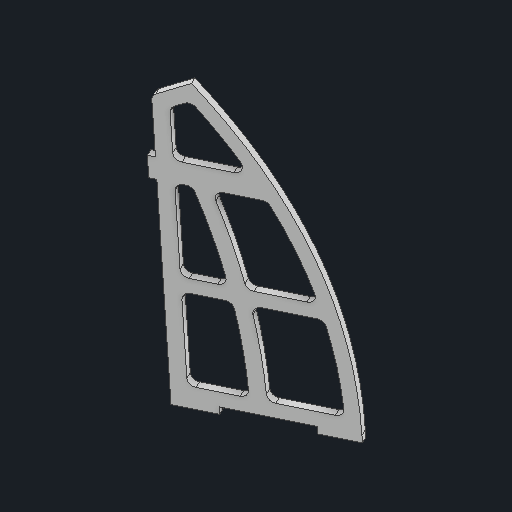
# Autodesk Inventor part: sponson_spanner_bottom
Saved by Autodesk Inventor 2022.2 (Build 262287010, 287A)
## iProperties
Created: 2022-03-22
Part Number: sponson_spanner_bottom
Material: Generic
Document SubType Name: Modeling
Designer: kardo
Density: 1 g/cm^3
Appearance: Default
Mass: 2.79206 g
Surface Area: 40.129 cm^2
Volume: 2.79206 cm^3
Author: kardo
Autodesk Inventor part; units mm, degrees
ref_plane "YZ Plane" through (0, 0, 0) normal (1, 0, 0) x (0, 1, 0)
ref_plane "XZ Plane" through (0, 0, 0) normal (0, 1, 0) x (-1, 0, 0)
ref_plane "XY Plane" through (0, 0, 0) normal (0, 0, 1) x (1, 0, 0)
derived "parameters_frame.ipt"
derived "stencil_frame.ipt"
sketch "sk_joint_locations" plane through (81.12, 0, 0) normal (1, 0, 0) x (0, 1, 0)
  line L0 (0, 0) -> (135.09, 9.4464) construction
  line L1 (30.81, 28.832) -> (94.8, 28.832) construction
  arc A0 (30.81, 28.832) -> (9.48, 28.4869) centre (30.81, -630.4631) ccw construction
  line L2 (-254.1001, 19.9549) -> (9.48, 28.4869) construction
  line L3 (-363, 18.496) -> (-275.8801, 19.4795) construction
  arc A1 (-275.8801, 19.4795) -> (-254.1001, 19.9549) centre (-287.5515, 1053.3708) ccw construction
  line L4 (25.1322, 1581.9163) -> (267.6663, -1886.4825) construction
  line L5 (-242.0001, 1541.8302) -> (-242.0001, -1877.3857) construction
  line L6 (-120.9999, 1541.8302) -> (-120.9999, -1877.3857) construction
  line L7 (-363, 1541.8302) -> (-363, -1877.3857) construction
  line L8 (0, 1541.8302) -> (0, -1877.3857) construction
  line L9 (450.0665, 43.8884) -> (-613.9211, 6.7332) construction
  line L10 (-677.4829, -27.4989) -> (501.7293, 54.9597) construction
  line L11 (187.7215, 30.7247) -> (187.4423, 38.7198) construction
  line L12 (195.4031, 37.5588) -> (195.9625, 29.5588) construction
  line L13 (0, 3.808) -> (134.9306, 11.7256) construction
  line L14 (-242.0001, 45.8501) -> (-242.0001, 20.3465) construction
  line L15 (-363, 37.4293) -> (-363, 18.496) construction
  line L16 (-120.9999, 51.0063) -> (-120.9999, 24.2633) construction
  line L17 (0, 52.89) -> (0, 28.18) construction
  line L18 (132.2944, 49.425) -> (132.8217, 41.8851) construction
  line L19 (133.3489, 34.3453) -> (132.8217, 41.8851) construction
  line L20 (133.3489, 34.3453) -> (133.8761, 26.8054) construction
  line L21 (133.8761, 26.8054) -> (134.4034, 19.2655) construction
  line L22 (134.4034, 19.2655) -> (134.9306, 11.7256) construction
  line L23 (0, 3.808) -> (0, 0) construction
  line L24 (94.8, 37.536) -> (94.8, 28.832) construction
  line L25 (94.8, 35.548) -> (94.8, 30.82) construction
  spline S0 degree 4 poles (-363, 37.4293) (-272.3626, 45.1427) (-181.5879, 49.7528) (-90.8131, 52.89) (0, 52.89) knots 0 0 0 0 0 1 1 1 1 1
  spline S1 degree 3 poles (0, 52.89) (86.3106, 52.89) (181.3207, 49.5034) (237, 36.448) knots 0 0 0 0 1 1 1 1
  spline S2 degree 2 poles (135.09, 9.4464) (188.144, 13.1563) (237, 36.448) knots 0 0 0 1 1 1
  point P0 (187.5819, 34.7223)
  point P1 (195.6828, 33.5588)
  point P2 (134.9575, 11.3411)
  point P3 (-363, 27.9627)
  point P4 (-242.0001, 33.0983)
  point P5 (-120.9999, 37.6348)
  point P6 (0, 40.535)
  point P7 (94.8, 33.184)
sketch "sk_spanner_joints_locations" plane through (0, 135.09, 9.4464) normal (0, 0.9975641, 0.0697565) x (-1, 0, 0)
  line L0 (266.3539, 10.2816) -> (-340.3092, 33.2601) construction
  line L1 (-958.4738, -367.3533) -> (724.0529, 375.1534) construction
  line L2 (-86.9102, 23.6621) -> (-85.7837, 17.7688) construction
  line L3 (-86.9102, 23.6621) -> (-73.574, 23.157) construction
  line L4 (-85.7837, 17.7688) -> (-73.574, 23.157) construction
  point P0 (0, 0)
  point P1 (-126.048, 0)
  point P2 (-156, 26.279)
  point P3 (-142.182, 25.7557)
  point P4 (-100.7281, 24.1855)
  point P5 (-95.8498, 13.3266)
  point P6 (-115.9819, 4.4422)
ref_plane "plane_strnger_outer" through (84.12, 0, 0) normal (1, 0, 0) x (0, 1, 0)
sketch "sk_corner_offset" plane through (0, 135.09, 9.4464) normal (0, 0.9975641, 0.0697565) x (-1, 0, 0)
  line L0 (-156, 26.279) -> (-126.048, 0) construction
  line L1 (-126.048, 0) -> (-81.12, 0) construction
  point P0 (0, 0)
  point P1 (-125.5962, 1.2)
  dimension "d7" = 1.2
  dimension "d8" = 1.2
  constraints: 4 end point, 1 horizontal
  measures "d7" distance from line of L0 point (-125.596, 1.2)
  measures "d8" distance from line of point (-125.596, 1.2) L1
sketch "sk_tip_offset" plane through (81.12, 0, 0) normal (1, 0, 0) x (0, 1, 0)
  spline S0 degree 3 poles (0, 52.89) (86.3106, 52.89) (181.3207, 49.5034) (237, 36.448) knots 0 0 0 0 1 1 1 1 construction
  spline S1 degree 2 poles (135.09, 9.4464) (188.144, 13.1563) (237, 36.448) knots 0 0 0 1 1 1 construction
  spline S2 degree 5 poles (0, 51.69) (13.1181, 51.69) (26.2363, 51.6248) (39.354, 51.4874) (65.3463, 51.0551) (91.3298, 50.254) (104.1978, 49.754) (128.8047, 48.5691) (153.3792, 46.8416) (165.0971, 45.8705) (185.8514, 43.8357) (206.5158, 41.0381) (215.5021, 39.6373) (224.4562, 38.0172) (233.3343, 36.0522) knots 0 0 0 0 0 0 0.280033 0.280033 0.280033 0.55492 0.55492 0.55492 0.805891 0.805891 0.805891 1 1 1 1 1 1
  spline S3 degree 5 poles (135.0063, 10.6435) (155.3816, 12.0688) (175.6301, 15.3217) (195.5215, 20.4957) (214.7957, 27.4783) (233.3343, 36.0523) knots 0 0 0 0 0 0 1 1 1 1 1 1
  point P0 (0, 0)
  dimension "d9" = 1.2
  dimension "d10" = 1.2
  constraints: 1 coincident, 6 other
sketch "sk_spanner_bottom_base" plane through (126.048, 0, 0) normal (0.4037383, -0.0638184, 0.9126459) x (-0.1841621, 0.9714748, 0.1494022)
  spline S0 degree 2 poles (132.6478, -27.2597) (191.4823, -39.3504) (243.959, 0) knots 0 0 0 1 1 1 construction
  line L0 (-538.2742, 157.4046) -> (483.8461, -52.6455) projected
  line L1 (132.8286, -26.3803) -> (130.8695, -25.9777)
  line L2 (130.8695, -25.9777) -> (132.9036, -16.0796)
  line L3 (132.9036, -16.0796) -> (134.8627, -16.4822)
  line L4 (134.8627, -16.4822) -> (139.2923, 5.0727)
  line L5 (139.2923, 5.0727) -> (137.3332, 5.4753)
  line L6 (137.3332, 5.4753) -> (139.548, 16.2527)
  line L7 (139.548, 16.2527) -> (141.5071, 15.8501)
  line L8 (141.5071, 15.8501) -> (141.8732, 17.6314)
  line L9 (132.6478, -27.2597) -> (0, 0) construction
  spline S1 degree 2 poles (132.8286, -26.3803) (189.8211, -38.0925) (240.3388, 0.6867) knots 0 0 0 1 1 1
  point P0 (23.2133, 112.9576)
  point P1 (132.6478, -27.2597)
  point P2 (203.3887, 8.3374)
  point P3 (240.3871, -2.6136)
  point P4 (0, 0)
  point P5 (236.8915, -1.8953)
  dimension "d4" = 2
  constraints: 16 end point, 3 parallel, 2 collinear, 2 perpendicular, 1 point on line, 5 other
  measures "d4" distance between parallel lines of L6 L4
extrude "thicken" add sketch "sk_spanner_bottom_base" along normal blind 2
sketch "sk_cut_weight" plane through (126.048, 0, 0) normal (0.4037383, -0.0638184, 0.9126459) x (-0.1841621, 0.9714748, 0.1494022)
  spline S0 degree 2 poles (132.8286, -26.3803) (189.8211, -38.0925) (240.3388, 0.6867) knots 0 0 0 1 1 1 construction
  line L0 (-538.2742, 157.4046) -> (483.8461, -52.6455) projected
  line L1 (134.8627, -16.4822) -> (139.2923, 5.0727) construction
  line L2 (141.5071, 15.8501) -> (141.8732, 17.6314) projected
  line L3 (203.3887, 8.3374) -> (196.9665, -22.9134) construction
  line L4 (141.5071, 15.8501) -> (198.4444, 4.1493)
  line L5 (198.4444, 4.1493) -> (198.8105, 5.9305)
  line L6 (204.6877, 4.7228) -> (204.3216, 2.9415)
  line L7 (204.3216, 2.9415) -> (236.5255, -3.6765)
  line L8 (144.62, 11.1268) -> (197.6392, 0.2312)
  line L9 (197.6392, 0.2312) -> (196.8257, -3.7273)
  line L10 (144.62, 11.1268) -> (141.8099, -2.5476)
  line L11 (203.5164, -0.9766) -> (200.0143, -18.0182)
  line L12 (236.5255, -3.6765) -> (236.8915, -1.8953)
  spline S1 degree 2 poles (137.0775, -5.7048) (168.2346, -12.1077) (200.1776, -7.288) knots 0 0 0 1 1 1
  line L13 (203.5164, -0.9766) -> (225.2505, -5.4431)
  line L14 (195.9736, -7.8742) -> (193.4279, -20.2614)
  line L15 (141.0045, -6.4667) -> (137.4844, -23.5958)
  line L16 (173.0887, 5.2764) -> (170.9056, -5.3466)
  line L17 (169.1706, 6.0816) -> (166.8413, -5.2526)
  line L18 (170.0858, -9.3358) -> (166.8204, -25.2254)
  line L19 (166.0249, -9.2253) -> (162.6946, -25.431)
  line L20 (171.1296, 5.679) -> (164.7537, -25.3467) construction
  line L21 (220.4235, -0.3675) -> (230.7941, -31.5659)
  line L22 (217.3562, -3.8208) -> (219.1113, -9.1006)
  line L23 (236.5255, -3.6765) -> (230.7941, -31.5659)
  spline S2 degree 5 poles (137.4844, -23.5958) (143.8697, -24.7118) (150.323, -25.4388) (156.8186, -25.7409) (170.5324, -25.4236) (184.0583, -23.0915) (191.0656, -21.3039) (202.345, -17.5012) (213.0997, -12.4377) (217.2427, -10.2649) (221.2933, -7.9283) (225.2505, -5.4431) knots 0 0 0 0 0 0 0.35312 0.35312 0.35312 0.745441 0.745441 0.745441 1 1 1 1 1 1
  spline S3 degree 5 poles (137.8827, -1.7867) (143.6031, -2.9621) (149.3718, -3.9026) (155.1771, -4.5995) (161.0049, -5.0491) (166.8413, -5.2526) knots 0 0 0 0 0 0 1 1 1 1 1 1
  spline S4 degree 5 poles (166.8413, -5.2526) (172.8495, -5.4621) (178.8668, -5.4107) (184.8781, -5.0995) (190.8684, -4.5348) (196.8257, -3.7273) knots 0 0 0 0 0 0 1 1 1 1 1 1
  point P0 (23.2133, 112.9576)
  point P1 (170.9056, -5.3466)
  dimension "d11" = 3.6057
  dimension "d17" = 4
  dimension "d12" = 2
  dimension "d13" = 4
  dimension "d14" = 4
  dimension "d15" = 4
  dimension "d18" = 4
  dimension "d22" = 60
  dimension "d23" = 4
  constraints: 43 end point, 9 collinear, 7 point on line, 6 parallel, 5 perpendicular, 4 midpoint, 29 other
  measures "d12" distance between parallel lines of L6 L3
  measures "d13" distance between parallel lines of L3 L5
  measures "d14" distance between parallel lines of L4 L8
  measures "d15" distance between parallel lines of L1 L10
  measures "d18" distance between parallel lines of L17 L16
  measures "d22" angle of L7 L21
  measures "d23" distance between parallel lines of L22 L21
extrude "cut_weight" cut sketch "sk_cut_weight" along normal through all both and the other way through all contours L0 L5 L4 L2 | L0 L12 L7 L6 | L23 L21 S2 L13 L7 | L13 S2 L21 | L22 S2 L11 L13 | L8 L17 S3 L10 | L8 L9 S4 L16 | S1 L19 S2 L15 | S1 L14 S2 L18
fillet "rounding" radius 2 21 edges at (89.8469, 197.8703, 30.9469) (89.8469, 166.8824, 28.78) (103.4947, 167.3025, 22.7718) (106.2791, 138.3954, 19.5187) (89.8469, 137.8896, 26.7526) (89.8469, 162.8921, 28.501) (104.1435, 163.3322, 22.2072) (89.8469, 191.8849, 30.5283) (97.4172, 192.118, 27.1957) (93.5441, 191.9987, 28.9007) (108.9868, 192.4741, 22.1024) (119.2795, 163.7982, 15.5439) (100.433, 163.218, 23.8406) (105.7637, 198.3603, 23.9398) (118.3354, 167.7594, 16.2385) (122.2776, 138.8879, 12.4757) (99.7687, 167.1878, 24.4121) (102.6187, 138.2828, 21.1301) (86.1874, 214.156, 33.7046) (89.8469, 211.9649, 31.9325) (94.2552, 214.8758, 30.1859)
equation "\"d7\" = shell_thickness"
equation "\"d8\" = shell_thickness"
equation "\"d9\" = shell_thickness"
equation "\"d10\" = shell_thickness"
equation "\"d4\" = bulkhead_thickness"
equation "\"d5\" = bulkhead_thickness"
equation "\"d17\" = bulkhead_inset"
equation "\"d12\" = bulkhead_thickness"
equation "\"d13\" = 2 * bulkhead_thickness"
equation "\"d14\" = bulkhead_inset"
equation "\"d15\" = bulkhead_inset"
equation "\"d18\" = bulkhead_inset"
equation "\"d23\" = bulkhead_inset"
equation "\"d21\" = 0.5 * bulkhead_inset"
equation "\"d3\" = stringer_thickness"
equation "\"shell_thickness\" = 1.2"
equation "\"bulkhead_thickness\" = 2"
equation "\"bulkhead_inset\" = 4"
equation "\"stringer_thickness\" = 3"
body "Solid1"
